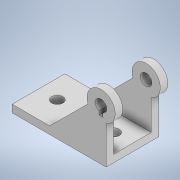
# Autodesk Inventor part: Top_Pulley_90
Saved by Autodesk Inventor 2020 (Build 240168000, 168)
## iProperties
Created: 2019-10-01
Part Number: Top_Pulley_90
Material: 일반
Document SubType Name: Modeling
Designer: Knowblesse
Density: 1 g/cm^3
Appearance: 기본값
Author: Knowblesse
## iProperties of the stored document _3D 인쇄.ipt
Created: 2019-10-01
Part Number: _3D 인쇄
Material: 일반
Document SubType Name: Modeling
Designer: Knowblesse
Density: 1 g/cm^3
Appearance: 기본값
Author: Knowblesse
Autodesk Inventor part; units mm, degrees
ref_plane "YZ Plane" through (0, 0, 0) normal (1, 0, 0) x (0, 1, 0)
ref_plane "XZ Plane" through (0, 0, 0) normal (0, 1, 0) x (-1, 0, 0)
ref_plane "XY Plane" through (0, 0, 0) normal (0, 0, 1) x (1, 0, 0)
sketch "스케치1" plane through (0, 0, 0) normal (0, 0, 1) x (1, 0, 0)
  line L0 (0, 0) -> (30, 30)
  line L1 (30, 30) -> (30, 0)
  line L2 (30, 0) -> (0, 0)
  circle A0 centre (27.3117, 22.9984) radius 7.5
  circle A1 centre (27.3117, 22.9984) radius 3.05
  point P0 (30, 15.9967)
  point P1 (20.3101, 20.3101)
  dimension "d2" = 15
  dimension "d0" = 30
  dimension "d1" = 30
  dimension "d3" = 6.1
  constraints: 6 end point, 1 centre point, 1 coincident, 1 perpendicular, 1 tangent, 1 vertical, 3 other
  measures "d0" distance of L0.end L1.end
  measures "d1" distance of L1.end L0.start
  measures "d3" diameter of A1
extrude "돌출1" add sketch "스케치1" along normal blind 4 contours L0 A0 L1 L2 | A0 L0 | L0 A1 L1 A0 | L0 L1 A1 | A0 L1 A1
sketch "스케치2" plane through (0, 0, 0) normal (0, -1, 0) x (1, 0, 0)
  line L0 (0, 0) -> (30, 0) projected
  line L1 (30, 0) -> (-20, 0)
  line L2 (-20, 0) -> (-20, 14)
  line L3 (-20, 14) -> (30, 14)
  line L4 (30, 14) -> (30, 0)
  dimension "d6" = 50
  dimension "d7" = 14
  constraints: 8 end point, 2 parallel, 1 horizontal, 1 perpendicular
  measures "d6" distance of L2.end L3.end
  measures "d7" distance between parallel lines of L3 L1
extrude "돌출2" add sketch "스케치2" along normal blind 4
mirror "미러1" about plane through (30, 0, 14) normal (0, 0, 1) of "돌출1", "돌출2"
sketch "스케치3" plane through (0, 0, 0) normal (0, 1, 0) x (1, 0, 0)
  line L0 (30, -4) -> (30, -24) construction
  line L1 (30, -14) -> (-20, -14) construction
  line L2 (-20, 0) -> (-20, -28) construction
  point P0 (0, 0)
  point P1 (-10, -14)
  point P2 (20, -14)
  dimension "d10" = 10
  dimension "d11" = 10
  constraints: 2 end point, 2 midpoint, 2 point on line
  measures "d10" distance from line of point (20, -14) L0
  measures "d11" distance from line of L2 point (-10, -14)
hole "구멍1" at (-10, 0, 14) at (20, 0, 14) direction (0, -1, 0) diameter 6 end through all
sketch "스케치4" plane through (-20, 0, 28) normal (0, 0, 1) x (1, 0, 0)
  circle A0 centre (47.3117, 22.9984) radius 3.05 projected
  line L0 (46.3117, 20.1984) -> (48.3117, 20.1984)
  line L1 (48.3117, 20.1984) -> (48.3117, 18.1984)
  line L2 (48.3117, 18.1984) -> (46.3117, 18.1984)
  line L3 (46.3117, 18.1984) -> (46.3117, 20.1984)
  point P0 (20, 0)
  point P1 (47.3117, 20.1984)
  point P2 (48.3117, 20.1169)
  point P3 (46.3117, 20.1169)
  dimension "d19" = 2
  dimension "d20" = 2
  dimension "d21" = 2.8
  constraints: 8 end point, 2 parallel, 1 horizontal, 1 midpoint, 1 perpendicular, 1 vertical alignment
  measures "d19" distance of L1.end L2.end
  measures "d20" distance of L0.end L1.end
  measures "d21" distance of A0.centre point (47.312, 20.198)
extrude "돌출3" cut sketch "스케치4" against normal blind 4 contours A0 L1 L2 L3
